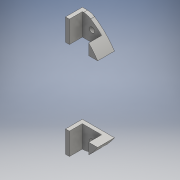
# Autodesk Inventor part: Left Standoff Support
Saved by Autodesk Inventor 2016 (Build 200138000, 138)
## iProperties
Created: 2017-03-16
Part Number: Left Standoff Support
Material: Generic
Document SubType Name: Modeling
Designer: Billy
Density: 1 g/cm^3
Appearance: Default
Author: Billy
Autodesk Inventor part; units mm, degrees
ref_plane "YZ Plane" through (0, 0, 0) normal (1, 0, 0) x (0, 1, 0)
ref_plane "XZ Plane" through (0, 0, 0) normal (0, 1, 0) x (-1, 0, 0)
ref_plane "XY Plane" through (0, 0, 0) normal (0, 0, 1) x (1, 0, 0)
sketch "Sketch1" plane through (0, 0, 0) normal (0, 1, 0) x (-1, 0, 0)
  arc A0 (-44.3621, -29) -> (-28.9848, -44.3721) centre (0, 0) ccw
  arc A1 (-28.9848, -44.3721) -> (-23.516, -46) centre (-23.516, -36) ccw
  line L0 (-23.516, -46) -> (-22.5467, -46)
  circle A2 centre (-30, -37.5) radius 2
  line L1 (-22.5467, -37.5) -> (-22.5467, -46)
  line L2 (-22.5467, -29) -> (-44.3621, -29)
  line L3 (-22.5467, -29) -> (-19.5467, -29)
  line L4 (-19.5467, -29) -> (-19.5467, -46)
  line L5 (-19.5467, -46) -> (-22.5467, -46)
  line L6 (0, 0) -> (-2.4935, 0)
  arc A3 (-28.9848, 44.3721) -> (-44.3621, 29) centre (0, 0) ccw
  line L7 (-23.516, 46) -> (-22.5467, 46)
  arc A4 (-23.516, 46) -> (-28.9848, 44.3721) centre (-23.516, 36) ccw
  circle A5 centre (-30, 37.5) radius 2
  line L8 (-22.5467, 37.5) -> (-22.5467, 46)
  line L9 (-22.5467, 29) -> (-44.3621, 29)
  line L10 (-22.5467, 29) -> (-19.5467, 29)
  line L11 (-19.5467, 29) -> (-19.5467, 46)
  line L12 (-19.5467, 46) -> (-22.5467, 46)
  dimension "d0" = 3
  constraints: 26 end point, 11 symmetric about line, 8 point on circle, 6 centre point, 3 horizontal, 2 perpendicular, 1 parallel, 3 other
  measures "d0" distance of L4.end L0.end
extrude "Extrusion1" add sketch "Sketch1" along normal blind 13
sketch "Sketch2" plane through (0, 0, 0) normal (0, -1, 0) x (1, 0, 0)
  circle A0 centre (30, 37.5) radius 2
  arc A1 (44.3621, 29) -> (28.9848, 44.3721) centre (0, 0) ccw
  arc A2 (28.9848, 44.3721) -> (23.516, 46) centre (23.516, 36) ccw
  line L0 (19.5467, 46) -> (23.516, 46)
  line L1 (19.5467, 29) -> (19.5467, 46)
  line L2 (44.3621, 29) -> (19.5467, 29)
  line L3 (44.3621, 29) -> (19.5467, 29) projected
  line L4 (19.5467, 46) -> (22.5467, 46)
  line L5 (22.5467, 46) -> (22.5467, 29)
  line L6 (22.5467, 29) -> (19.5467, 29)
  line L7 (19.5467, 29) -> (19.5467, 46)
  line L8 (37.4533, 37.5) -> (37.4533, 29)
  line L9 (0, 0) -> (2.6946, 0)
  circle A3 centre (30, -37.5) radius 2
  arc A4 (28.9848, -44.3721) -> (44.3621, -29) centre (0, 0) ccw
  arc A5 (23.516, -46) -> (28.9848, -44.3721) centre (23.516, -36) ccw
  line L10 (19.5467, -46) -> (23.516, -46)
  line L11 (19.5467, -29) -> (19.5467, -46)
  line L12 (44.3621, -29) -> (19.5467, -29)
  line L13 (44.3621, -29) -> (19.5467, -29)
  line L14 (19.5467, -46) -> (22.5467, -46)
  line L15 (22.5467, -46) -> (22.5467, -29)
  line L16 (22.5467, -29) -> (19.5467, -29)
  line L17 (19.5467, -29) -> (19.5467, -46)
  line L18 (37.4533, -37.5) -> (37.4533, -29)
  dimension "d3" = 3
  constraints: 36 end point, 12 symmetric about line, 10 centre point, 10 point on circle, 4 point on line, 2 horizontal, 2 parallel, 1 perpendicular, 1 vertical, 3 other
  measures "d3" distance of L1.start L5.end
extrude "Extrusion2" cut sketch "Sketch2" against normal blind 10 contours L8 L2 L5 L0 A2 A1 | A5 L10 L15 L12 L18 A4
body "Solid1"
